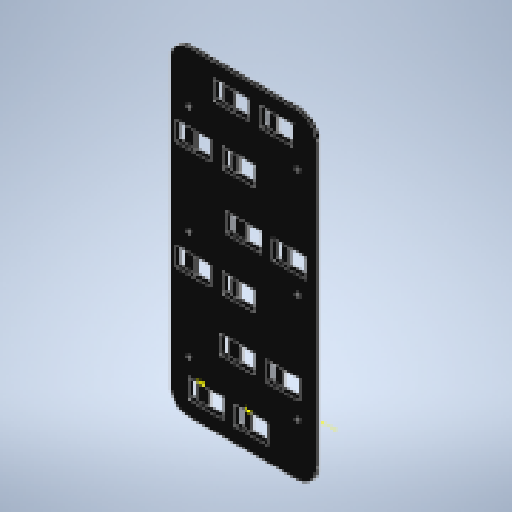
# Autodesk Inventor part: backplate-0
Saved by Autodesk Inventor 2024.1 (Build 281209000, 209)
## iProperties
Created: 2024-09-24
Part Number: backplate-0
Material: Generic
Document SubType Name: Modeling
Designer: Imogen Heard
Density: 1 g/cm^3
Appearance: Glossy - Black
Author: Imogen Heard
Autodesk Inventor part; units mm, degrees
ref_plane "YZ Plane" through (0, 0, 0) normal (1, 0, 0) x (0, 1, 0)
ref_plane "Work Plane1" through (2.7698, 1, -3.5) normal (0, 0, 1) x (1, 0, 0)
sketch "Sketch15" plane through (0, 0, 0) normal (0, 1, 0) x (-1, 0, 0)
  line L0 (-25.7706, -0.5) -> (-39.1567, -0.5)
  arc A0 (-28.2201, -1.5) -> (-25.7706, -0.5) centre (-28.2201, 2) ccw
  line L1 (-39.056, -1.5) -> (-28.2201, -1.5)
  arc A1 (-39.056, -1.5) -> (-40.256, -2.7) centre (-39.056, -2.7) ccw
  line L2 (-40.256, -2.8) -> (-40.256, -2.7)
  arc A2 (-40.256, -2.8) -> (-39.056, -4) centre (-39.056, -2.8) ccw
  arc A3 (-2.1567, -0.5) -> (-9.5221, -4) centre (-2.1567, -10) ccw
  line L3 (11.2294, -0.5) -> (-2.1567, -0.5)
  arc A4 (8.7799, -1.5) -> (11.2294, -0.5) centre (8.7799, 2) ccw
  line L4 (-2.056, -1.5) -> (8.7799, -1.5)
  arc A5 (-2.056, -1.5) -> (-3.256, -2.7) centre (-2.056, -2.7) ccw
  line L5 (-3.256, -4.5) -> (-3.256, -2.7)
  line L6 (-46.9026, -4.5) -> (-63.8013, -4.5)
  line L7 (12.044, -9.6962) -> (12.044, -4.5)
  line L8 (-4.8746, -39) -> (12.044, -9.6962)
  line L9 (-19.3953, -43.5) -> (-12.6688, -43.5)
  line L10 (-19.3953, -42.5) -> (-19.3953, -43.5)
  line L11 (-12.3801, -42.5) -> (-19.3953, -42.5)
  line L12 (10.7139, -10) -> (-5.8849, -38.75)
  arc A6 (10.7139, -10) -> (8.1158, -5.5) centre (8.1158, -8.5) ccw
  line L13 (-64.09, -5.5) -> (8.1158, -5.5)
  line L14 (-84.8746, -34) -> (-70.5852, -9.25)
  arc A7 (-92.6688, -38.5) -> (-84.8746, -34) centre (-92.6688, -29.5) ccw
  line L15 (-104.3953, -38.5) -> (-92.6688, -38.5)
  line L16 (-104.3953, -37.5) -> (-104.3953, -38.5)
  line L17 (-71.5955, -9) -> (-85.8849, -33.75)
  line L18 (-39.1567, 0) -> (-24.756, 0)
  arc A8 (-28.2201, -2) -> (-24.756, 0) centre (-28.2201, 2) ccw
  arc A9 (-28.0636, -2.4575) -> (-25.2561, -1.7034) centre (-26.756, -1.7224) ccw
  line L19 (-28.2201, -2) -> (-39.056, -2)
  line L20 (11.2294, -0.5) -> (-2.1567, -0.5)
  line L21 (-2.1567, -0.5) -> (-2.1567, 0)
  line L22 (-2.1567, 0) -> (12.244, 0)
  spline S0 degree 3 poles (11.2294, -0.5) (11.5862, -0.3543) (11.9249, -0.1842) (12.244, 0) knots 0 0 0 0 1 1 1 1
  arc A10 (-2.1567, 0) -> (-9.756, -3.5) centre (-2.1567, -10) ccw
  arc A11 (8.7799, -2) -> (12.244, 0) centre (8.7799, 2) ccw
  arc A12 (8.9364, -2.4575) -> (11.7439, -1.7034) centre (10.244, -1.7224) ccw
  line L23 (8.7799, -2) -> (-2.056, -2)
  line L24 (-39.056, -3.5) -> (-28.1636, -3.5)
  line L25 (-28.1636, -3.5) -> (-28.1636, -2)
  line L26 (-28.1636, -2) -> (-40.7028, -2)
  line L27 (-24.4636, 0.5) -> (-17.356, 0.5)
  line L28 (-17.356, 0.5) -> (-17.356, -3.5)
  line L29 (-24.4636, -3.5) -> (-24.4636, 0.5)
  line L30 (-2.056, -2) -> (8.8364, -2)
  line L31 (8.8364, -2) -> (8.8364, -3.5)
  line L32 (8.8364, -3.5) -> (-2.056, -3.5)
  line L33 (12.5364, 0.5) -> (16.5364, 0.5)
  line L34 (16.5364, 0.5) -> (16.5364, -3.5)
  line L35 (16.5364, -3.5) -> (12.5364, -3.5)
  line L36 (12.5364, -3.5) -> (12.5364, 0.5)
  line L37 (-54.356, 0.5) -> (-58.356, 0.5)
  line L38 (-58.356, 0.5) -> (-58.356, -3.5)
  line L39 (-58.356, -3.5) -> (-54.356, -3.5)
  line L40 (-54.356, -3.5) -> (-54.356, 0.5)
  line L41 (-54.356, 0) -> (-43.356, 0)
  line L42 (-43.356, 0) -> (-43.356, 0.5)
  line L43 (-43.356, 0.5) -> (-54.356, 0.5)
  line L44 (-54.356, 0.5) -> (-54.356, 0)
  line L45 (-17.356, 0.5) -> (-6.356, 0.5)
  line L46 (-6.356, 0.5) -> (-6.356, 0)
  line L47 (-6.356, 0) -> (-17.356, 0)
  line L48 (-17.356, 0) -> (-17.356, 0.5)
  line L49 (-9.5221, -4) -> (-39.056, -4)
  line L50 (-24.4636, -3.5) -> (-17.356, -3.5)
  line L51 (-35.056, -3.5) -> (-35.056, -2)
  line L52 (-1.556, -3.5) -> (-1.556, -2)
  arc A13 (-39.1567, -0.5) -> (-46.9026, -4.5) centre (-39.1567, -10) ccw
  line L53 (12.044, -4.5) -> (-3.256, -4.5)
  arc A14 (-12.6688, -43.5) -> (-4.8746, -39) centre (-12.6688, -34.5) ccw
  arc A15 (-12.3801, -42.5) -> (-5.8849, -38.75) centre (-12.3801, -35) ccw
  arc A16 (-64.09, -5.5) -> (-70.5852, -9.25) centre (-64.09, -13) ccw
  line L54 (-92.3801, -37.5) -> (-104.3953, -37.5)
  arc A17 (-92.3801, -37.5) -> (-85.8849, -33.75) centre (-92.3801, -30) ccw
  arc A18 (-63.8013, -4.5) -> (-71.5955, -9) centre (-63.8013, -13.5) ccw
  point P0 (0, 0)
  point P1 (-37.9028, -4)
  point P2 (11.2206, -4.5)
  point P3 (16.5364, -1.5)
  point P4 (-28.1636, -2.75)
  point P5 (-1.556, -2)
  point P6 (-35.056, -2)
  point P7 (-43.356, 0.25)
  dimension "d143" = 14.4007
  dimension "d147" = 4
  dimension "d149" = 3.7
  dimension "d151" = 4
  dimension "d152" = 4
  dimension "d154" = 11
  dimension "d155" = 11
  dimension "d162" = 3.7
  dimension "d163" = 7.1076
  dimension "d174" = 4
  dimension "d175" = 0.5
  dimension "d176" = 4.1993
  dimension "d177" = 4.1993
  dimension "d178" = 0.1
  dimension "d179" = 0.1
  constraints: 56 end point, 11 parallel, 8 horizontal, 8 horizontal alignment, 7 perpendicular, 7 point on line, 3 midpoint, 2 vertical, 1 coincident, 1 vertical alignment
  measures "d143" distance of L22.end L21.end
  measures "d147" distance from line of point (16.536, -1.5) L36
  measures "d149" distance between parallel lines of L36 L31
  measures "d151" distance between parallel lines of L33 L35
  measures "d152" distance between parallel lines of L38 L40
  measures "d154" distance between parallel lines of L42 L40
  measures "d155" distance between parallel lines of L46 L28
  measures "d162" distance from line of point (-28.164, -2.75) L29
  measures "d163" distance between parallel lines of L28 L29
  measures "d174" distance from line of L51 A2.centre
  measures "d175" distance from line of A5.centre L52
  measures "d176" horizontal distance of L18.start point (-43.356, 0.25)
  measures "d177" distance from line of L21.end L46
  measures "d178" distance from line of L31 A12.start
  measures "d179" distance from line of L25 A9.start
extrude "Extrusion12" add sketch "Sketch15" along normal blind 15.2 contours A8 L25 L24 L51 L19 | A11 L31 L32 L52 L23 | L27 L28 L50 L29 | L33 L34 L35 L36 | L40 L39 L38 L37
sketch "Sketch16" plane through (0, 0, 0) normal (0, -1, 0) x (1, 0, 0)
  line L0 (58.356, -3.5) -> (54.356, -3.5) projected
  line L1 (-16.5364, -3.5) -> (-16.5364, 0.5) projected
  line L2 (58.356, -3.5) -> (-16.5364, -3.5)
  line L3 (-16.5364, -3.5) -> (-16.5364, 0.5)
  line L4 (-16.5364, 0.5) -> (58.356, 0.5)
  line L5 (58.356, 0.5) -> (58.356, -3.5)
  point P0 (0, 0)
  constraints: 8 end point, 2 parallel, 1 horizontal, 1 perpendicular
extrude "Extrusion13" add sketch "Sketch16" along normal blind 2
sketch "Sketch17" plane through (0, 15.2, 0) normal (0, 1, 0) x (1, 0, 0)
  line L0 (58.356, -0.5) -> (-16.5364, -0.5) projected
  line L1 (-16.5364, -0.5) -> (-16.5364, 3.5) projected
  line L2 (-16.5364, 3.5) -> (58.356, 3.5) projected
  line L3 (58.356, 3.5) -> (58.356, -0.5) projected
  point P0 (0, 0)
extrude "Extrusion14" add sketch "Sketch17" along normal blind 2
sketch "Sketch14" plane through (-13.1974, 17.2, 0) normal (0, 1, 0) x (1, 0, 0)
  line L0 (84.7183, 18.5) -> (62.0935, 4.9251) construction
  line L1 (84.7183, 18.5) -> (98.331, 18.5) construction
  line L2 (98.331, 20.5) -> (98.331, 18.5) construction
  line L3 (88.6008, 20.5) -> (98.331, 20.5) construction
  arc A0 (88.6008, 20.5) -> (83.9703, 19.2174) centre (88.6008, 11.5) ccw construction
  line L4 (63.7206, 7.0676) -> (83.9703, 19.2174) construction
  arc A1 (58.0611, 5.5) -> (63.7206, 7.0676) centre (58.0611, 16.5) ccw construction
  line L5 (10.0711, 5.5) -> (58.0611, 5.5) construction
  arc A2 (7.9497, 10.6213) -> (10.0711, 5.5) centre (10.0711, 8.5) ccw construction
  line L6 (16.8284, 19.5) -> (7.9497, 10.6213) construction
  line L7 (23.5, 19.5) -> (16.8284, 19.5) construction
  line L8 (23.5, 20.5) -> (23.5, 19.5) construction
  line L9 (16.4142, 20.5) -> (23.5, 20.5) construction
  line L10 (4, 8.0858) -> (16.4142, 20.5) construction
  line L11 (4, 4.5) -> (4, 8.0858) construction
  line L12 (30.1619, 4.5) -> (4, 4.5) construction
  line L13 (30.1619, 2.7) -> (30.1619, 4.5) construction
  arc A3 (28.9619, 1.5) -> (30.1619, 2.7) centre (28.9619, 2.7) ccw construction
  line L14 (13.4641, 1.5) -> (28.9619, 1.5) construction
  arc A4 (13.4641, 1.5) -> (11.0146, 0.5) centre (13.4641, -2) ccw construction
  line L15 (29.0626, 0.5) -> (11.0146, 0.5) construction
  arc A5 (29.0626, 0.5) -> (36.428, 4) centre (29.0626, 10) ccw construction
  line L16 (53.9619, 4) -> (36.428, 4) construction
  arc A6 (55.1619, 2.8) -> (53.9619, 4) centre (53.9619, 2.8) ccw construction
  line L17 (55.1619, 2.7) -> (55.1619, 2.8) construction
  arc A7 (53.9619, 1.5) -> (55.1619, 2.7) centre (53.9619, 2.7) ccw construction
  line L18 (50.126, 1.5) -> (53.9619, 1.5) construction
  arc A8 (50.126, 1.5) -> (47.6765, 0.5) centre (50.126, -2) ccw construction
  line L19 (54.0626, 0.5) -> (47.6765, 0.5) construction
  arc A9 (54.0626, 0.5) -> (62.0935, 4.9251) centre (54.0626, 10) ccw construction
  line L20 (10, 0) -> (29.0626, 0) construction
  arc A10 (13.4641, 2) -> (10, 0) centre (13.4641, -2) ccw construction
  line L21 (28.9619, 2) -> (13.4641, 2) construction
  arc A11 (28.9619, 2) -> (29.6619, 2.7) centre (28.9619, 2.7) ccw construction
  line L22 (29.6619, 4) -> (29.6619, 2.7) construction
  line L23 (4, 4.5) -> (30.1619, 4.5) construction
  line L24 (4, 4.5) -> (30.1619, 4.5) construction
  line L25 (53.9619, 2) -> (50.126, 2) construction
  arc A12 (50.126, 2) -> (46.6619, 0) centre (50.126, -2) ccw construction
  arc A13 (54.0626, 0) -> (62.4513, 4.5567) centre (54.0626, 10) ccw construction
  arc A14 (61.6619, 3.5) -> (62.4513, 4.5567) centre (54.0626, 10) ccw construction
  line L26 (61.6619, 3.5) -> (86.6619, 18.5) construction
  line L27 (86.6619, 18.5) -> (84.7183, 18.5) construction
  line L28 (84.7183, 18.5) -> (62.0935, 4.9251) construction
  spline S0 degree 2 poles (62.4513, 4.5567) (62.2707, 4.7438) (62.0935, 4.9251) knots 0 0 0 1 1 1 weights 1 1 1 construction
  spline S1 degree 3 poles (11.4805, 2.4087) (11.2979, 2.2729) (11.1516, 2.1215) (10.9661, 1.9036) (10.9068, 1.8279) (10.757, 1.6898) (10.6546, 1.6468) (10.3427, 1.5246) (10.1265, 1.4295) (9.9146, 1.2822) knots 0 0 0 0 0.267596 0.267596 0.445672 0.445672 0.696555 0.696555 1 1 1 1 construction
  arc A15 (11.4805, 2.4087) -> (9.9146, 1.2822) centre (11.1619, 1.2) ccw construction
  spline S2 degree 3 poles (12.2519, 1.8119) (12.2417, 1.8319) (12.2264, 1.8618) (12.1362, 1.9854) (12.0877, 2.0448) (11.973, 2.1534) (11.9138, 2.2025) (11.7896, 2.2826) (11.7353, 2.3126) (11.6138, 2.3675) (11.5482, 2.3909) (11.4805, 2.4087) knots 0 0 0 0 0.361956 0.361956 0.597365 0.597365 0.7682 0.7682 0.881321 0.881321 1 1 1 1 construction
  spline S3 degree 3 poles (10.2353, 0.3611) (10.2253, 0.3714) (10.2105, 0.387) (10.1432, 0.4739) (10.1051, 0.5275) (10.039, 0.648) (10.0097, 0.7087) (9.9605, 0.8483) (9.9408, 0.9205) (9.9133, 1.0915) (9.9083, 1.186) (9.9146, 1.2822) knots 0 0 0 0 0.295028 0.295028 0.533101 0.533101 0.699955 0.699955 0.841987 0.841987 1 1 1 1 construction
  arc A16 (48.068, 2.4023) -> (46.476, 1.2084) centre (47.726, 1.2) ccw construction
  spline S4 degree 3 poles (46.476, 1.2084) (46.4754, 1.1138) (46.4856, 1.0216) (46.5219, 0.8547) (46.5453, 0.7842) (46.602, 0.6471) (46.6349, 0.5874) (46.7092, 0.4683) (46.7516, 0.4153) (46.8273, 0.3288) (46.8442, 0.3133) (46.8555, 0.303) knots 0 0 0 0 0.152523 0.152523 0.291399 0.291399 0.457448 0.457448 0.697801 0.697801 1 1 1 1 construction
  spline S5 degree 3 poles (48.8309, 1.7845) (48.8207, 1.8059) (48.8053, 1.8379) (48.7137, 1.9688) (48.6639, 2.0319) (48.5469, 2.145) (48.4878, 2.195) (48.3654, 2.2756) (48.3129, 2.3054) (48.196, 2.3602) (48.1331, 2.3838) (48.068, 2.4023) knots 0 0 0 0 0.368463 0.368463 0.609666 0.609666 0.778405 0.778405 0.88683 0.88683 1 1 1 1 construction
ref_plane "Work Plane2" through (-9.1974, 15, -20.5) normal (0, 1, 0) x (0, 0, 1)
chamfer "Chamfer10" distance 1 angle 45 2 edges at (35.056, 7.6, -2) (1.556, 7.6, -2)
sketch "Sketch18" plane through (0, 15.2, 0) normal (0, -1, 0) x (1, 0, 0)
  line L0 (17.356, 0.5) -> (15.356, 0.5)
  line L1 (15.356, 0.5) -> (15.356, -3.5)
  line L2 (15.356, -3.5) -> (17.356, -3.5)
  line L3 (17.356, -3.5) -> (17.356, 0.5)
  line L4 (54.356, 0.5) -> (50.356, 0.5)
  line L5 (50.356, 0.5) -> (50.356, -3.5)
  line L6 (50.356, -3.5) -> (54.356, -3.5)
  line L7 (54.356, -3.5) -> (54.356, 0.5)
  point P0 (0, 0)
  dimension "d167" = 4
  dimension "d168" = 2
  constraints: 16 end point, 6 coincident, 4 parallel, 2 horizontal, 2 perpendicular
  measures "d167" distance between parallel lines of L5 L7
  measures "d168" distance between parallel lines of L1 L3
extrude "Extrusion15" add sketch "Sketch18" along normal blind 15.2
chamfer "Chamfer11" distance 2 angle 45 2 edges at (50.356, 7.6, -3.5) (15.356, 7.6, -3.5)
sketch "Sketch6" plane through (-1.4016, 0, 0.5) normal (0, 0, 1) x (1, 0, 0)
  line L0 (51.7576, 15.2) -> (51.7576, 0) projected
  line L1 (51.7576, 0) -> (25.8652, 0) projected
  line L2 (25.8652, 0) -> (25.8652, 15.2) projected
  line L3 (25.8652, 15.2) -> (51.7576, 15.2) projected
  line L4 (59.7576, -2) -> (59.7576, 17.2) projected
  line L5 (-15.1348, 17.2) -> (59.7576, 17.2) projected
  line L6 (-15.1348, -2) -> (-15.1348, 17.2) projected
  line L7 (59.7576, -2) -> (-15.1348, -2) projected
  line L8 (-11.1348, 15.2) -> (16.7576, 15.2) projected
  line L9 (16.7576, 15.2) -> (16.7576, 0) projected
  line L10 (16.7576, 0) -> (-11.1348, 0) projected
  line L11 (-11.1348, 0) -> (-11.1348, 15.2) projected
extrude "Extrusion5" add sketch "Sketch6" along normal blind 0.5
sketch "Sketch7" plane through (-1.4016, 0, 1) normal (0, 0, 1) x (1, 0, 0)
  line L0 (79.8429, 232) -> (4.9505, 232)
  line L1 (4.9505, 232) -> (4.9505, 212.8)
  line L2 (4.9505, 212.8) -> (79.8429, 212.8)
  line L3 (79.8429, 212.8) -> (79.8429, 232)
  line L4 (49.7576, 189) -> (-25.1348, 189)
  line L5 (-25.1348, 189) -> (-25.1348, 169.8)
  line L6 (-25.1348, 169.8) -> (49.7576, 169.8)
  line L7 (49.7576, 169.8) -> (49.7576, 189)
  line L8 (14.8652, 146) -> (14.8652, 126.8)
  line L9 (89.7576, 146) -> (14.8652, 146)
  line L10 (14.8652, 126.8) -> (89.7576, 126.8)
  line L11 (89.7576, 126.8) -> (89.7576, 146)
  line L12 (9.8652, 60) -> (9.8652, 40.8)
  line L13 (84.7576, 60) -> (9.8652, 60)
  line L14 (9.8652, 40.8) -> (84.7576, 40.8)
  line L15 (84.7576, 40.8) -> (84.7576, 60)
  line L16 (-25.1348, 103) -> (-25.1348, 83.8)
  line L17 (49.7576, 83.8) -> (49.7576, 103)
  line L18 (-25.1348, 83.8) -> (49.7576, 83.8)
  line L19 (49.7576, 103) -> (-25.1348, 103)
  line L20 (59.7576, -2) -> (59.7576, 17.2) projected
  line L21 (59.7576, 17.2) -> (-15.1348, 17.2) projected
  line L22 (-15.1348, 17.2) -> (-15.1348, -2) projected
  line L23 (-15.1348, -2) -> (59.7576, -2) projected
  line L24 (51.7576, 15.2) -> (51.7576, 0) projected
  line L25 (51.7576, 0) -> (25.8652, 0) projected
  line L26 (25.8652, 0) -> (25.8652, 15.2) projected
  line L27 (25.8652, 15.2) -> (51.7576, 15.2) projected
  line L28 (-11.1348, 15.2) -> (16.7576, 15.2) projected
  line L29 (16.7576, 15.2) -> (16.7576, 0) projected
  line L30 (16.7576, 0) -> (-11.1348, 0) projected
  line L31 (-11.1348, 0) -> (-11.1348, 15.2) projected
  line L32 (84.7576, 60) -> (84.7576, 382.798) construction
  point P0 (52.3114, 146)
  point P1 (42.3967, 232)
  dimension "d58" = 19.2
  dimension "d66" = 19.2
  dimension "d72" = 19.2
  dimension "d74" = 19.2
  dimension "d81" = 43
  dimension "d82" = 43
  dimension "d83" = 43
  dimension "d84" = 43
  dimension "d180" = 19.2
  dimension "d181" = 74.8924
  dimension "d182" = 42.8
  dimension "d183" = 74.8924
  dimension "d184" = 74.8924
  dimension "d185" = 25
  dimension "d186" = 10
  dimension "d187" = 74.8924
  dimension "d188" = 74.8924
  dimension "d189" = 74.8924
  dimension "d190" = 19.2
  dimension "d197" = 30
  constraints: 42 end point, 10 parallel, 5 coincident, 5 horizontal, 5 perpendicular, 2 midpoint, 2 vertical alignment, 1 vertical
  measures "d58" distance between parallel lines of L2 L0
  measures "d66" distance between parallel lines of L10 L9
  measures "d72" distance between parallel lines of L14 L13
  measures "d74" distance between parallel lines of L18 L19
  measures "d81" distance between parallel lines of L4 L0
  measures "d82" distance between parallel lines of L9 L4
  measures "d83" distance from line of L19 point (52.311, 146)
  measures "d84" distance between parallel lines of L13 L19
  measures "d180" distance between parallel lines of L23 L21
  measures "d181" distance between parallel lines of L22 L20
  measures "d182" distance between parallel lines of L21 L13
  measures "d183" distance between parallel lines of L12 L15
  measures "d184" distance between parallel lines of L16 L17
  measures "d185" distance between parallel lines of L15 L20
  measures "d186" distance between parallel lines of L22 L16
  measures "d187" distance between parallel lines of L1 L3
  measures "d188" distance between parallel lines of L5 L7
  measures "d189" distance between parallel lines of L8 L11
  measures "d190" distance between parallel lines of L6 L4
  measures "d197" distance between parallel lines of L11 L20
pattern_sketch "Sketch Driven Pattern1" from (58.356, 17.2, 1) copies at (78.4413, 232, 1) at (48.356, 189, 1) at (88.356, 146, 1) at (48.356, 103, 1) at (83.356, 60, 1)
sketch "Sketch8" plane through (-1.4016, 0, 1) normal (0, 0, 1) x (1, 0, 0)
  line L0 (-25.6348, -2) -> (90.3652, -2)
  line L1 (90.3652, -2) -> (90.3652, 242)
  line L2 (-25.6348, 194.4422) -> (-25.6348, -2)
  line L3 (-15, -2) -> (56.6619, -2)
  line L4 (90.3652, -2) -> (-25.6348, -2)
  line L5 (-25.6348, -2) -> (-25.6348, -12)
  line L6 (-25.6348, -12) -> (90.3652, -12)
  line L7 (90.3652, -12) -> (90.3652, -2)
  line L8 (-25.6348, 127.957) -> (-25.6348, 242)
  line L9 (-25.6348, 242) -> (90.3652, 242)
  line L10 (-25.1348, 103) -> (-25.1348, 83.8) projected
  line L11 (-25.1348, 83.8) -> (-25.1348, 103) projected
  line L12 (89.7576, 126.8) -> (89.7576, 146) projected
  line L13 (59.7576, -2) -> (59.7576, 17.2) projected
  line L14 (-15.1348, -2) -> (59.7576, -2) projected
  line L15 (-15.1348, -2) -> (-15.1348, 17.2) projected
  line L16 (59.7576, 17.2) -> (-15.1348, 17.2) projected
  line L17 (-11.1348, 0) -> (-11.1348, 15.2) projected
  line L18 (-11.1348, 0) -> (-7.4348, 0) projected
  line L19 (-7.4348, 0) -> (-7.4348, 15.2) projected
  line L20 (-7.4348, 15.2) -> (-11.1348, 15.2) projected
  line L21 (2.9576, 0) -> (18.7576, 0) projected
  line L22 (18.7576, 15.2) -> (18.7576, 0) projected
  line L23 (18.7576, 15.2) -> (2.9576, 15.2) projected
  line L24 (2.9576, 0) -> (2.9576, 15.2) projected
  line L25 (36.4576, 0) -> (53.7576, 0) projected
  line L26 (53.7576, 15.2) -> (53.7576, 0) projected
  line L27 (29.5652, 15.2) -> (25.8652, 15.2) projected
  line L28 (25.8652, 0) -> (25.8652, 15.2) projected
  line L29 (-25.1348, 169.8) -> (49.7576, 169.8) projected
  line L30 (-25.1348, 169.8) -> (-25.1348, 189) projected
  line L31 (49.7576, 189) -> (-25.1348, 189) projected
  line L32 (-25.1348, 169.8) -> (49.7576, 169.8) projected
  line L33 (51.7576, 0) -> (51.7576, 15.2) projected
  line L34 (16.7576, 0) -> (16.7576, 15.2) projected
  line L35 (53.7576, 15.2) -> (36.4576, 15.2) projected
  line L36 (36.4576, 0) -> (36.4576, 15.2) projected
  line L37 (25.8652, 0) -> (29.5652, 0) projected
  line L38 (29.5652, 0) -> (29.5652, 15.2) projected
  line L39 (84.7576, 40.8) -> (84.7576, 60) projected
  line L40 (9.8652, 40.8) -> (84.7576, 40.8) projected
  line L41 (9.8652, 40.8) -> (9.8652, 60) projected
  line L42 (84.7576, 60) -> (9.8652, 60) projected
  line L43 (13.8652, 42.8) -> (13.8652, 58) projected
  line L44 (13.8652, 42.8) -> (17.5652, 42.8) projected
  line L45 (17.5652, 42.8) -> (17.5652, 58) projected
  line L46 (17.5652, 58) -> (13.8652, 58) projected
  line L47 (61.4576, 42.8) -> (78.7576, 42.8) projected
  line L48 (78.7576, 58) -> (78.7576, 42.8) projected
  line L49 (78.7576, 58) -> (61.4576, 58) projected
  line L50 (61.4576, 42.8) -> (61.4576, 58) projected
  line L51 (27.9576, 42.8) -> (43.7576, 42.8) projected
  line L52 (43.7576, 58) -> (43.7576, 42.8) projected
  line L53 (43.7576, 58) -> (27.9576, 58) projected
  line L54 (27.9576, 42.8) -> (27.9576, 58) projected
  line L55 (54.5652, 58) -> (50.8652, 58) projected
  line L56 (50.8652, 42.8) -> (50.8652, 58) projected
  line L57 (50.8652, 42.8) -> (54.5652, 42.8) projected
  line L58 (54.5652, 42.8) -> (54.5652, 58) projected
  line L59 (89.7576, 126.8) -> (89.7576, 146) projected
  line L60 (14.8652, 126.8) -> (89.7576, 126.8) projected
  line L61 (14.8652, 126.8) -> (14.8652, 146) projected
  line L62 (89.7576, 146) -> (14.8652, 146) projected
  line L63 (18.8652, 128.8) -> (18.8652, 144) projected
  line L64 (18.8652, 128.8) -> (22.5652, 128.8) projected
  line L65 (22.5652, 128.8) -> (22.5652, 144) projected
  line L66 (22.5652, 144) -> (18.8652, 144) projected
  line L67 (66.4576, 128.8) -> (83.7576, 128.8) projected
  line L68 (83.7576, 144) -> (83.7576, 128.8) projected
  line L69 (83.7576, 144) -> (66.4576, 144) projected
  line L70 (66.4576, 128.8) -> (66.4576, 144) projected
  line L71 (32.9576, 128.8) -> (48.7576, 128.8) projected
  line L72 (48.7576, 144) -> (48.7576, 128.8) projected
  line L73 (48.7576, 144) -> (32.9576, 144) projected
  line L74 (32.9576, 128.8) -> (32.9576, 144) projected
  line L75 (59.5652, 144) -> (55.8652, 144) projected
  line L76 (55.8652, 128.8) -> (55.8652, 144) projected
  line L77 (55.8652, 128.8) -> (59.5652, 128.8) projected
  line L78 (59.5652, 128.8) -> (59.5652, 144) projected
  line L79 (49.7576, 83.8) -> (49.7576, 103) projected
  line L80 (-25.1348, 83.8) -> (49.7576, 83.8) projected
  line L81 (-25.1348, 83.8) -> (-25.1348, 103) projected
  line L82 (49.7576, 103) -> (-25.1348, 103) projected
  line L83 (-21.1348, 85.8) -> (-21.1348, 101) projected
  line L84 (-21.1348, 85.8) -> (-17.4348, 85.8) projected
  line L85 (-17.4348, 85.8) -> (-17.4348, 101) projected
  line L86 (-17.4348, 101) -> (-21.1348, 101) projected
  line L87 (26.4576, 85.8) -> (43.7576, 85.8) projected
  line L88 (43.7576, 101) -> (43.7576, 85.8) projected
  line L89 (43.7576, 101) -> (26.4576, 101) projected
  line L90 (26.4576, 85.8) -> (26.4576, 101) projected
  line L91 (-7.0424, 85.8) -> (8.7576, 85.8) projected
  line L92 (8.7576, 101) -> (8.7576, 85.8) projected
  line L93 (8.7576, 101) -> (-7.0424, 101) projected
  line L94 (-7.0424, 85.8) -> (-7.0424, 101) projected
  line L95 (19.5652, 101) -> (15.8652, 101) projected
  line L96 (15.8652, 85.8) -> (15.8652, 101) projected
  line L97 (15.8652, 85.8) -> (19.5652, 85.8) projected
  line L98 (19.5652, 85.8) -> (19.5652, 101) projected
  line L99 (49.7576, 169.8) -> (49.7576, 189) projected
  line L100 (-25.1348, 169.8) -> (49.7576, 169.8) projected
  line L101 (-25.1348, 169.8) -> (-25.1348, 189) projected
  line L102 (49.7576, 189) -> (-25.1348, 189) projected
  line L103 (-21.1348, 171.8) -> (-21.1348, 187) projected
  line L104 (-21.1348, 171.8) -> (-17.4348, 171.8) projected
  line L105 (-17.4348, 171.8) -> (-17.4348, 187) projected
  line L106 (-17.4348, 187) -> (-21.1348, 187) projected
  line L107 (26.4576, 171.8) -> (43.7576, 171.8) projected
  line L108 (43.7576, 187) -> (43.7576, 171.8) projected
  line L109 (43.7576, 187) -> (26.4576, 187) projected
  line L110 (26.4576, 171.8) -> (26.4576, 187) projected
  line L111 (-7.0424, 171.8) -> (8.7576, 171.8) projected
  line L112 (8.7576, 187) -> (8.7576, 171.8) projected
  line L113 (8.7576, 187) -> (-7.0424, 187) projected
  line L114 (-7.0424, 171.8) -> (-7.0424, 187) projected
  line L115 (19.5652, 187) -> (15.8652, 187) projected
  line L116 (15.8652, 171.8) -> (15.8652, 187) projected
  line L117 (15.8652, 171.8) -> (19.5652, 171.8) projected
  line L118 (19.5652, 171.8) -> (19.5652, 187) projected
  line L119 (79.8429, 212.8) -> (79.8429, 232) projected
  line L120 (4.9505, 212.8) -> (79.8429, 212.8) projected
  line L121 (4.9505, 212.8) -> (4.9505, 232) projected
  line L122 (79.8429, 232) -> (4.9505, 232) projected
  line L123 (8.9505, 214.8) -> (8.9505, 230) projected
  line L124 (8.9505, 214.8) -> (12.6505, 214.8) projected
  line L125 (12.6505, 214.8) -> (12.6505, 230) projected
  line L126 (12.6505, 230) -> (8.9505, 230) projected
  line L127 (56.5429, 214.8) -> (73.8429, 214.8) projected
  line L128 (73.8429, 230) -> (73.8429, 214.8) projected
  line L129 (73.8429, 230) -> (56.5429, 230) projected
  line L130 (56.5429, 214.8) -> (56.5429, 230) projected
  line L131 (23.0429, 214.8) -> (38.8429, 214.8) projected
  line L132 (38.8429, 230) -> (38.8429, 214.8) projected
  line L133 (38.8429, 230) -> (23.0429, 230) projected
  line L134 (23.0429, 214.8) -> (23.0429, 230) projected
  line L135 (49.6505, 230) -> (45.9505, 230) projected
  line L136 (45.9505, 214.8) -> (45.9505, 230) projected
  line L137 (45.9505, 214.8) -> (49.6505, 214.8) projected
  line L138 (49.6505, 214.8) -> (49.6505, 230) projected
  point P0 (1.4016, 0)
  point P1 (-25.6348, -2)
  point P2 (59.7576, -2)
  dimension "d97" = 254
  dimension "d193" = 116
  dimension "d194" = 0.5
  dimension "d208" = 10
  dimension "d209" = 10
  constraints: 18 end point, 3 parallel, 2 horizontal, 2 perpendicular, 1 coincident, 1 horizontal alignment, 1 point on line
  measures "d97" distance between parallel lines of L9 L6
  measures "d193" distance between parallel lines of L2 L1
  measures "d194" distance between parallel lines of L2 L10
  measures "d208" distance between parallel lines of L9 L122
  measures "d209" distance between parallel lines of L6 L0
extrude "Extrusion6" add sketch "Sketch8" against normal up to surface (4.5 mm away) contours L2 L8 L9 L1 L0 L13 L16 L15 | L0 L7 L6 L5
fillet "Fillet2" radius 15 4 edges at (-27.0364, -12, -1.25) (88.9636, -12, -1.25) (-27.0364, 242, -1.25) (88.9636, 242, -1.25)
chamfer "Chamfer7" distance 5 distance2 2 7 edges at (-22.643, -7.6066, -3.5) (30.9636, -12, -3.5) (84.5702, -7.6066, -3.5) (88.9636, 115, -3.5) (84.5702, 237.6066, -3.5) (30.9636, 242, -3.5) (-22.643, 237.6066, -3.5)
sketch "Sketch9" plane through (64.4445, 237, -3.5) normal (0, 0, -1) x (-1, 0, 0)
  circle A0 centre (-9.519, -207.8) radius 1.55
  circle A1 centre (76.481, -207.8) radius 1.55
  circle A2 centre (76.481, -36) radius 1.55
  circle A3 centre (-9.519, -36) radius 1.55
  circle A4 centre (-9.519, -122) radius 1.55
  circle A5 centre (76.481, -122) radius 1.55
  line L0 (91.481, -234) -> (91.481, -10) projected
  line L1 (83.281, -136) -> (49.981, -136) projected
  line L2 (-24.519, -10) -> (-24.519, -234) projected
  line L3 (12.0885, -221.8) -> (39.981, -221.8) projected
  line L4 (83.281, -50) -> (49.981, -50) projected
  line L5 (-9.519, -249) -> (76.481, -249) projected
  line L6 (76.481, 5) -> (-9.519, 5) projected
  point P0 (64.4445, -237)
  point P1 (22.0885, -136)
  point P2 (22.0885, -50)
  dimension "d101" = 3.1
  dimension "d198" = 15
  dimension "d199" = 14
  dimension "d200" = 15
  dimension "d201" = 14
  dimension "d203" = 14
  dimension "d204" = 41.2
  dimension "d205" = 41
  dimension "d206" = 127
  dimension "d207" = 127
  constraints: 6 centre point, 5 equal radius, 4 vertical alignment, 3 horizontal alignment
  measures "d101" diameter of A0
  measures "d198" distance from line of L0 A1.centre
  measures "d199" distance from line of L1 A4.centre
  measures "d200" distance from line of L2 A0.centre
  measures "d201" distance from line of A0.centre L3
  measures "d203" distance from line of A3.centre L4
  measures "d204" distance from line of A1.centre L5
  measures "d205" distance from line of A2.centre L6
  measures "d206" distance from line of L6 A5.centre
  measures "d207" distance from line of A5.centre L5
extrude "Extrusion7" cut sketch "Sketch9" against normal through all
chamfer "Chamfer8" distance 3 angle 45 6 edges at (-10.4864, 115, -3.5) (75.5136, 115, -3.5) (75.5136, 201, -3.5) (-10.4864, 201, -3.5) (75.5136, 29.2, -3.5) (-10.4864, 29.2, -3.5)
equation "\"d81\" = d88"
equation "\"d82\" = d88"
equation "\"d83\" = d88"
equation "\"d84\" = d88"
equation "\"d88\" = 43"
body "Solid2"
